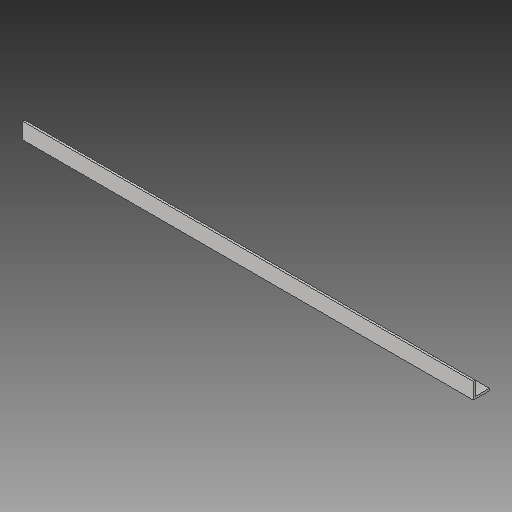
# Autodesk Inventor part: Aluminum L channel guard rail
Saved by Autodesk Inventor 2019 (Build 230136000, 136)
## iProperties
Created: 2019-03-18
Part Number: Aluminum L channel guard rail
Material: Generic
Document SubType Name: Modeling
Designer: josh
Density: 1 g/cm^3
Appearance: Default
Mass: 48.178 g
Surface Area: 408.257 cm^2
Volume: 48.178 cm^3
Author: josh
Autodesk Inventor part; units mm, degrees
ref_plane "YZ Plane" through (0, 0, 0) normal (1, 0, 0) x (0, 1, 0)
ref_plane "XZ Plane" through (0, 0, 0) normal (0, 1, 0) x (-1, 0, 0)
ref_plane "XY Plane" through (0, 0, 0) normal (0, 0, 1) x (1, 0, 0)
sketch "Sketch1" plane through (0, 0, 0) normal (1, 0, 0) x (0, 1, 0)
  line L0 (0, 0) -> (0, -19.05)
  line L1 (0, -19.05) -> (2.54, -19.05)
  line L2 (0, 0) -> (19.05, 0)
  line L3 (19.05, 0) -> (19.05, -2.54)
  line L4 (19.05, -2.54) -> (2.54, -2.54)
  line L5 (2.54, -2.54) -> (2.54, -19.05)
  dimension "d0" = 19.05
  dimension "d1" = 2.54
  dimension "d2" = 19.05
  dimension "d3" = 2.54
  constraints: 12 end point, 4 perpendicular, 1 horizontal, 1 vertical
  measures "d0" distance of L0.start L0.end
  measures "d1" distance of L0.end L1.end
  measures "d2" distance of L0.start L2.end
  measures "d3" distance of L2.end L3.end
extrude "Extrusion1" add sketch "Sketch1" along normal blind 533.4
body "Solid1"
